output_shaft_thread v3 (Autodesk Fusion 360 design; units mm, degrees)
Autodesk Fusion 360 part; units mm, degrees
note: some values were not read from the file. Set by a fixed rule: which sketch regions a step uses.
sketch "Sketch1" plane through (0, 0, 0) normal (0, 0, 1) x (1, 0, 0)
  circle A0 centre (0, 0) radius 9
  circle A1 centre (0, 0) radius 16 construction
  line L0 (0, 0) -> (0, 16) construction
  circle A2 centre (0, 16) radius 3.5
  circle A3 centre (-15.2169, 4.9443) radius 3.5
  circle A4 centre (-9.4046, -12.9443) radius 3.5
  circle A5 centre (9.4046, -12.9443) radius 3.5
  circle A6 centre (15.2169, 4.9443) radius 3.5
  circle A7 centre (0, 0) radius 15
  circle A8 centre (0, 0) radius 21
  circle A9 centre (0, 0) radius 12 construction
  line L1 (0, 0) -> (-8.8168, 12.1353) construction
  circle A10 centre (-7.0534, 9.7082) radius 2
  circle A11 centre (-7.0534, 9.7082) radius 2.25 construction
  circle A12 centre (-11.4127, -3.7082) radius 2
  circle A13 centre (0, -12) radius 2
  circle A14 centre (11.4127, -3.7082) radius 2
  circle A15 centre (7.0534, 9.7082) radius 2
  line L2 (0, 0) -> (-15.2169, 4.9443) construction
  circle A16 centre (0, 16) radius 2.25
  circle A17 centre (-15.2169, 4.9443) radius 2.25
  circle A18 centre (-9.4046, -12.9443) radius 2.25
  circle A19 centre (9.4046, -12.9443) radius 2.25
  circle A20 centre (15.2169, 4.9443) radius 2.25
  circle A21 centre (0, 0) radius 8.5
  dimension "d1" = 18
  dimension "d3" = 7
  dimension "d5" = 360
  dimension "d6" = 30
  dimension "d7" = 42
  dimension "d8" = 4
  dimension "d9" = 4.5
  dimension "d10" = 24
  dimension "d12" = 360
  dimension "d13" = 36
  dimension "d14" = 72
  dimension "d17" = 4.5
  dimension "d19" = 360
  dimension "d26" = 17
  dimension "d31" = 32
  constraint coincident A0.centre A1.centre
  constraint coincident A1 L0.end
  constraint vertical L0
  constraint coincident L0.end A2.centre
  constraint concentric A1 A8
  constraint concentric A8 A9
  constraint coincident A7 L1.end
  constraint coincident A9 A10.centre
  constraint coincident L1 A10.centre
  constraint concentric A10 A11
  constraint coincident A3.centre L2.end
  constraint concentric A2 A16
  constraint concentric A9 A21
  measures "d1" diameter of A0
  measures "d3" diameter of A2
  measures "d6" diameter of A7
  measures "d7" diameter of A8
  measures "d8" diameter of A10
  measures "d9" diameter of A11
  measures "d10" diameter of A9
  measures "d13" angle of L0 L1
  measures "d14" angle of L0 L2
  measures "d17" diameter of A16
  measures "d26" diameter of A21
  measures "d31" diameter of A1
extrude "Extrude1" add sketch "Sketch1" along normal blind 6 contours A2 A3 A4 A5 A6 A7 | A8
extrude "Extrude6" add sketch "Sketch1" along normal blind 14 contours A2 A3 A4 A5 A6 A7
extrude "Extrude7" add sketch "Sketch1" along normal blind 6 contours A2 A7 A16 | A2 A7 A16 | A3 A7 A17 | A3 A7 A17 | A6 A7 A20 | A6 A7 A20 | A4 A7 A18 | A4 A7 A18 | A5 A7 A19 | A5 A7 A19
extrude "Extrude4" add sketch "Sketch1" along normal blind 14 contours A0
extrude "Extrude5" cut sketch "Sketch1" along normal blind 4 contours A0
sketch "Sketch2" plane through (0, 0, 6) normal (0, 0, 1) x (-1, 0, 0)
  circle A0 centre (0, 0) radius 21
  arc A1 (-12.9338, -7.5971) -> (-3.2285, -14.6484) centre (0, 0) ccw
  arc A2 (-12.9338, -7.5971) -> (-14.9292, -1.4561) centre (-15.2169, -4.9443) ccw
  arc A3 (-11.2221, 9.9532) -> (-14.9292, -1.4561) centre (0, 0) ccw
  arc A4 (-11.2221, 9.9532) -> (-5.9982, 13.7485) centre (-9.4046, 12.9443) ccw
  arc A5 (5.9982, 13.7485) -> (-5.9982, 13.7485) centre (0, 0) ccw
  arc A6 (5.9982, 13.7485) -> (11.2221, 9.9532) centre (9.4046, 12.9443) ccw
  arc A7 (14.9292, -1.4561) -> (11.2221, 9.9532) centre (0, 0) ccw
  arc A8 (14.9292, -1.4561) -> (12.9338, -7.5971) centre (15.2169, -4.9443) ccw
  arc A9 (3.2285, -14.6484) -> (12.9338, -7.5971) centre (0, 0) ccw
  arc A10 (3.2285, -14.6484) -> (-3.2285, -14.6484) centre (0, -16) ccw
  circle A11 centre (0, 0) radius 17.5
  circle A12 centre (9.4046, 12.9443) radius 2.25
  circle A13 centre (15.2169, -4.9443) radius 2.25
  circle A14 centre (-9.4046, 12.9443) radius 2.25
  circle A15 centre (0, -16) radius 2.25
  circle A16 centre (-15.2169, -4.9443) radius 2.25
  dimension "d36" = 35
  constraint coincident A0.centre A1.centre
  measures "d36" diameter of A11
extrude "Extrude8" cut sketch "Sketch2" against normal blind 0.5 contours A0
sketch "Sketch3" plane through (0, 0, 0) normal (0, 0, -1) x (1, 0, 0)
  circle A0 centre (0, 0) radius 9
  circle A1 centre (-9.4046, 12.9443) radius 2.25
  circle A2 centre (-15.2169, -4.9443) radius 2.25
  circle A3 centre (9.4046, 12.9443) radius 2.25
  circle A4 centre (0, -16) radius 2.25
  circle A5 centre (15.2169, -4.9443) radius 2.25
  circle A6 centre (-7.0534, -9.7082) radius 2
  circle A7 centre (11.4127, 3.7082) radius 2
  circle A8 centre (0, 12) radius 2
  circle A9 centre (7.0534, -9.7082) radius 2
  circle A10 centre (-11.4127, 3.7082) radius 2
  circle A11 centre (0, 0) radius 21
extrude "Extrude9" add sketch "Sketch3" against normal blind 4 contours A6 | A7 | A8 | A9 | A10
equation "d10 = ( d6 - d1 ) / 2 + d1"
equation "d13 = d14 / 2"
